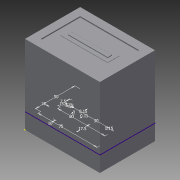
# Autodesk Inventor part: UMD_Gas_Burner
Saved by Autodesk Inventor 2013 SP2 (Build 170200200, 200)
## iProperties
Created: 2015-09-21
Part Number: UMD_Gas_Burner
Material: Generic
Document SubType Name: Modeling
Designer: mcgratta
Density: 1 g/cm^3
Author: mcgratta
Autodesk Inventor part; units mm, degrees
ref_plane "YZ Plane" through (0, 0, 0) normal (1, 0, 0) x (0, 1, 0)
ref_plane "XZ Plane" through (0, 0, 0) normal (0, 1, 0) x (-1, 0, 0)
ref_plane "XY Plane" through (0, 0, 0) normal (0, 0, 1) x (1, 0, 0)
sketch "Sketch1" plane through (0, 0, 0) normal (0, 1, 0) x (-1, 0, 0)
  point P0 (0, 0)
sketch "Sketch2" plane through (0, 0, 0) normal (0, 1, 0) x (-1, 0, 0)
  line L0 (0, 0) -> (-950, 0)
  line L1 (-950, 0) -> (-950, -700)
  line L2 (-950, -700) -> (0, -700)
  line L3 (0, -700) -> (0, 0)
  dimension "d0" = 700
  dimension "d2" = 950
  constraints: 8 end point, 2 parallel, 1 horizontal, 1 perpendicular
  measures "d0" distance between parallel lines of L0 L2
  measures "d2" distance between parallel lines of L1 L3
extrude "Extrusion1" add sketch "Sketch2" along normal blind 200
sketch "Sketch4" plane through (0, 200, 0) normal (0, 1, 0) x (1, 0, 0)
  line L0 (0, 0) -> (950, 0) projected
  line L1 (0, 700) -> (0, 0) projected
  line L2 (0, 0) -> (950, 0)
  line L3 (950, 0) -> (950, 700)
  line L4 (950, 700) -> (0, 700)
  line L5 (0, 700) -> (0, 0)
  line L6 (100, 100) -> (850, 100)
  line L7 (850, 100) -> (850, 600)
  line L8 (850, 600) -> (100, 600)
  line L9 (100, 600) -> (100, 100)
  line L10 (175, 275) -> (775, 275)
  line L11 (775, 275) -> (775, 425)
  line L12 (775, 425) -> (175, 425)
  line L13 (175, 425) -> (175, 275)
  line L14 (223.5, 323.5) -> (726.5, 323.5)
  line L15 (726.5, 323.5) -> (726.5, 376.5)
  line L16 (726.5, 376.5) -> (223.5, 376.5)
  line L17 (223.5, 376.5) -> (223.5, 323.5)
  line L18 (225, 325) -> (725, 325)
  line L19 (725, 325) -> (725, 375)
  line L20 (725, 375) -> (225, 375)
  line L21 (225, 375) -> (225, 325)
  dimension "d20" = 1.5
  dimension "d22" = 1.5
  dimension "d23" = 1.5
  dimension "d24" = 1.5
  dimension "d25" = 750
  dimension "d26" = 600
  dimension "d27" = 500
  dimension "d28" = 150
  dimension "d29" = 50
  dimension "d30" = 50
  dimension "d31" = 100
  dimension "d32" = 100
  dimension "d33" = 75
  dimension "d34" = 175
  dimension "d35" = 500
  dimension "d36" = 50
  constraints: 40 end point, 10 parallel, 5 horizontal, 5 perpendicular
  measures "d20" distance between parallel lines of L14 L18
  measures "d22" distance between parallel lines of L20 L16
  measures "d23" distance between parallel lines of L21 L17
  measures "d24" distance between parallel lines of L15 L19
  measures "d25" distance of L6.start L6.end
  measures "d26" distance of L10.start L10.end
  measures "d27" distance of L8.end L6.start
  measures "d28" distance of L12.end L10.start
  measures "d29" distance between parallel lines of L18 L10
  measures "d30" distance of L20.end L18.start
  measures "d31" distance between parallel lines of L0 L6
  measures "d32" distance between parallel lines of L1 L9
  measures "d33" distance between parallel lines of L9 L13
  measures "d34" distance between parallel lines of L6 L10
  measures "d35" distance between parallel lines of L19 L21
  measures "d36" distance between parallel lines of L13 L21
extrude "Extrusion3" add sketch "Sketch4" along normal blind 800 contours L17 L16 L15 L14
extrude "Extrusion4" add sketch "Sketch4" along normal blind 790 contours L13 L12 L11 L10
extrude "Extrusion5" add sketch "Sketch4" along normal blind 785 contours L9 L8 L7 L6
extrude "Extrusion6" add sketch "Sketch4" along normal blind 800 contours L1 L4 L3 L0
extrude "Extrusion7" add sketch "Sketch4" along normal blind 799 contours L21 L20 L19 L18
body "Solid1"
